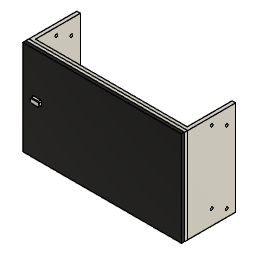
Radio Stack Avionics Template v10 (Autodesk Fusion 360 design; units mm, degrees)
Autodesk Fusion 360 part; units mm, degrees
sketch "Faceplate" plane through (0, 0, 0) normal (0, 1, 0) x (1, 0, 0) in component "Faceplate"
  line L0 (79.375, -47.3279) -> (-79.375, -47.3279)
  line L1 (-79.375, -47.3279) -> (-79.375, 47.3279)
  line L2 (-79.375, 47.3279) -> (79.375, 47.3279)
  line L3 (79.375, 47.3279) -> (79.375, -47.3279)
  line L4 (79.375, -47.3279) -> (-79.375, 47.3279) construction
  line L5 (-79.375, -47.3279) -> (79.375, 47.3279) construction
  line L6 (-65.5187, -6.373) -> (-65.5187, -0.373) construction
  arc A0 (-69.0187, -0.373) -> (-70.5187, -1.873) centre (-69.0187, -1.873) ccw
  line L7 (-62.0187, -0.373) -> (-69.0187, -0.373)
  line L8 (-70.5187, -1.873) -> (-70.5187, -4.873)
  line L9 (-60.5187, -4.873) -> (-60.5187, -1.873)
  arc A1 (-62.0187, -6.373) -> (-60.5187, -4.873) centre (-62.0187, -4.873) ccw
  line L10 (-69.0187, -6.373) -> (-62.0187, -6.373)
  arc A2 (-70.5187, -4.873) -> (-69.0187, -6.373) centre (-69.0187, -4.873) ccw
  arc A3 (-60.5187, -1.873) -> (-62.0187, -0.373) centre (-62.0187, -1.873) ccw
  line L11 (-77.2756, -49.1415) -> (67.16, -49.1415) construction
  line L12 (67.16, -49.1415) -> (67.16, -65.0937) construction
  line L13 (67.16, -65.0937) -> (-77.2756, -65.0937) construction
  line L14 (-77.2756, -65.0937) -> (-77.2756, -49.1415) construction
  point P0 (-65.5187, -3.373)
  dimension "d1" = 158.75
  dimension "d27" = 1.5
  dimension "d28" = 6
  dimension "d29" = 10
  dimension "d42" = 3
  constraint horizontal L0
  constraint perpendicular L0 L1
  constraint parallel L0 L2
  constraint parallel L1 L3
  constraint coincident L4 origin
  constraint coincident L5 origin
  constraint horizontal L10
  constraint vertical L9
  constraint horizontal L7
  constraint vertical L8
  constraint tangent A1 L10
  constraint tangent L9 A1
  constraint tangent L9 A3
  constraint tangent L7 A3
  constraint equal A1 A3
  constraint tangent A0 L7
  constraint tangent A0 L8
  constraint equal A0 A1
  constraint tangent L8 A2
  constraint tangent L10 A2
  constraint equal A1 A2
  constraint midpoint L6.start L10
  constraint midpoint L6.end L7
  constraint midpoint P0 L6
  measures "d1" distance of L1.end L2.end
  measures "d27" radius of A1
  measures "d28" distance of L7 L10
  measures "d29" distance of L8 L9
extrude "Extrude1" add sketch "Faceplate" against normal blind 3 makes body 1 in component "Faceplate"
ref_plane "WorkPlane1" through (0, 0, 0) normal (0, 1, 0) x (0, 0, 1) in component "Button Skirt Spacer"
sketch "Button Skirt (Gives buttons space behind faceplate)" plane through (0, 0, 0) normal (0, 1, 0) x (1, 0, 0) in component "Button Skirt Spacer"
  line L0 (-79.375, -47.3279) -> (-79.375, 47.3279)
  line L1 (79.375, -47.3279) -> (-79.375, -47.3279)
  line L2 (79.375, 47.3279) -> (79.375, -47.3279)
  line L3 (-79.375, 47.3279) -> (79.375, 47.3279)
  line L4 (-60.5187, -4.873) -> (-60.5187, -1.873)
  arc A0 (-62.0187, -6.373) -> (-60.5187, -4.873) centre (-62.0187, -4.873) ccw
  line L5 (-69.0187, -6.373) -> (-62.0187, -6.373)
  arc A1 (-70.5187, -4.873) -> (-69.0187, -6.373) centre (-69.0187, -4.873) ccw
  line L6 (-70.5187, -1.873) -> (-70.5187, -4.873)
  arc A2 (-69.0187, -0.373) -> (-70.5187, -1.873) centre (-69.0187, -1.873) ccw
  line L7 (-62.0187, -0.373) -> (-69.0187, -0.373)
  arc A3 (-60.5187, -1.873) -> (-62.0187, -0.373) centre (-62.0187, -1.873) ccw
  line L8 (-72.5187, -8.373) -> (-58.5187, -8.373)
  line L9 (-58.5187, -8.373) -> (-58.5187, 1.627)
  line L10 (-58.5187, 1.627) -> (-72.5187, 1.627)
  line L11 (-72.5187, 1.627) -> (-72.5187, -8.373)
  line L12 (-65.7771, -46.8251) -> (92.1912, -46.8251) construction
  line L13 (92.1912, -46.8251) -> (92.1912, -80.2756) construction
  line L14 (92.1912, -80.2756) -> (-65.7771, -80.2756) construction
  line L15 (-65.7771, -80.2756) -> (-65.7771, -46.8251) construction
  dimension "d37" = 2
  dimension "d38" = 2
  dimension "d39" = 2
  dimension "d40" = 2
  dimension "d41" = 3
  constraint horizontal L8
  constraint vertical L9
  constraint horizontal L10
  constraint vertical L11
  constraint horizontal L14
  measures "d37" distance of L4 L9
  measures "d38" distance of L5 L8
  measures "d39" distance of L6 L11
  measures "d40" distance of L7 L10
extrude "Extrude1'" add sketch "Button Skirt (Gives buttons space behind faceplate)" along normal blind 3 separate body contours L0 L1 L2 L3 | L4 A0 L5 A1 L6 A2 L7 A3 | L8 L9 L10 L11 makes body 2 in component "Button Skirt Spacer"
ref_plane "WorkPlane1" through (0, 3, 0) normal (0, 1, 0) x (0, 0, 1) in component "Non PCB Backing"
sketch "Sketch1" plane through (0, 3, 0) normal (0, 1, 0) x (1, 0, 0) in component "Non PCB Backing"
  line L0 (-79.375, -47.3279) -> (79.375, -47.3279)
  line L1 (-79.375, 47.3279) -> (-79.375, -47.3279)
  line L2 (79.375, 47.3279) -> (-79.375, 47.3279)
  line L3 (79.375, -47.3279) -> (79.375, 47.3279)
  arc A0 (-60.5187, -1.873) -> (-62.0187, -0.373) centre (-62.0187, -1.873) ccw construction
  line L4 (-62.0187, -0.373) -> (-69.0187, -0.373) construction
  arc A1 (-69.0187, -0.373) -> (-70.5187, -1.873) centre (-69.0187, -1.873) ccw construction
  line L5 (-70.5187, -1.873) -> (-70.5187, -4.873) construction
  arc A2 (-70.5187, -4.873) -> (-69.0187, -6.373) centre (-69.0187, -4.873) ccw construction
  line L6 (-69.0187, -6.373) -> (-62.0187, -6.373) construction
  arc A3 (-62.0187, -6.373) -> (-60.5187, -4.873) centre (-62.0187, -4.873) ccw construction
  line L7 (-60.5187, -4.873) -> (-60.5187, -1.873) construction
  line L8 (-79.375, 47.3279) -> (79.375, 47.3279)
  line L9 (79.375, 47.3279) -> (79.375, -47.3279)
  line L10 (79.375, -47.3279) -> (-79.375, -47.3279)
  line L11 (-79.375, -47.3279) -> (-79.375, 47.3279)
  line L12 (-69.0187, -4.873) -> (-62.0187, -1.873) construction
  line L13 (-62.4187, -0.123) -> (-68.6187, -0.123)
  line L14 (-68.6187, -0.123) -> (-68.6187, -6.623)
  line L15 (-68.6187, -6.623) -> (-62.4187, -6.623)
  line L16 (-62.4187, -6.623) -> (-62.4187, -0.123)
  line L17 (-62.4187, -0.123) -> (-68.6187, -6.623) construction
  line L18 (-68.6187, -0.123) -> (-62.4187, -6.623) construction
  line L19 (-152.6605, -47.3864) -> (11.8867, -47.2695) construction
  line L20 (11.8867, -47.2695) -> (11.9439, -127.8922) construction
  line L21 (11.9439, -127.8922) -> (-152.6032, -128.0091) construction
  line L22 (-152.6032, -128.0091) -> (-152.6605, -47.3864) construction
  line L23 (23.3274, -102.3824) -> (37.404, -102.3824)
  line L24 (37.404, -102.3824) -> (37.404, -92.7252)
  line L25 (37.404, -92.7252) -> (23.3274, -92.7252)
  line L26 (23.3274, -92.7252) -> (23.3274, -102.3824)
  line L27 (30.3657, -102.3824) -> (30.3657, -92.7252) construction
  line L28 (52.3764, -102.1676) -> (52.3764, -92.5104) construction
  line L29 (59.4147, -102.1676) -> (59.4147, -92.5104)
  line L30 (45.3381, -92.5104) -> (45.3381, -102.1676)
  line L31 (45.3381, -102.1676) -> (59.4147, -102.1676)
  line L32 (59.4147, -92.5104) -> (45.3381, -92.5104)
  line L33 (84.4147, -92.5104) -> (70.3381, -92.5104)
  line L34 (70.3381, -102.1676) -> (84.4147, -102.1676)
  line L35 (70.3381, -92.5104) -> (70.3381, -102.1676)
  line L36 (77.3764, -102.1676) -> (77.3764, -92.5104) construction
  line L37 (84.4147, -102.1676) -> (84.4147, -92.5104)
  line L38 (80.4764, -94.089) -> (74.2764, -94.089)
  line L39 (74.2764, -94.089) -> (74.2764, -100.589)
  line L40 (74.2764, -100.589) -> (80.4764, -100.589)
  line L41 (80.4764, -100.589) -> (80.4764, -94.089)
  line L42 (80.4764, -94.089) -> (74.2764, -100.589) construction
  line L43 (74.2764, -94.089) -> (80.4764, -100.589) construction
  line L44 (125.2683, -93.5274) -> (119.0683, -93.5274)
  line L45 (119.0683, -100.0274) -> (125.2683, -100.0274)
  line L46 (125.2683, -93.5274) -> (119.0683, -100.0274) construction
  line L47 (119.0683, -93.5274) -> (125.2683, -100.0274) construction
  line L48 (117.1683, -95.2774) -> (117.1683, -98.2774) construction
  arc A4 (118.6683, -93.7774) -> (117.1683, -95.2774) centre (118.6683, -95.2774) ccw construction
  line L49 (127.1683, -98.2774) -> (127.1683, -95.2774) construction
  line L50 (125.6683, -93.7774) -> (118.6683, -93.7774) construction
  arc A5 (127.1683, -95.2774) -> (125.6683, -93.7774) centre (125.6683, -95.2774) ccw construction
  arc A6 (125.6683, -99.7774) -> (127.1683, -98.2774) centre (125.6683, -98.2774) ccw construction
  arc A7 (117.1683, -98.2774) -> (118.6683, -99.7774) centre (118.6683, -98.2774) ccw construction
  line L51 (118.6683, -99.7774) -> (125.6683, -99.7774) construction
  line L52 (119.0683, -93.5274) -> (119.0683, -100.0274)
  line L53 (125.2683, -100.0274) -> (125.2683, -93.5274)
  line L54 (118.6683, -98.2774) -> (125.6683, -95.2774) construction
  line L55 (94.2764, -94.089) -> (94.2764, -100.589)
  line L56 (90.3381, -102.1676) -> (104.4147, -102.1676) construction
  line L57 (94.2764, -94.089) -> (100.4764, -100.589) construction
  line L58 (90.3381, -92.5104) -> (90.3381, -102.1676) construction
  line L59 (94.2764, -100.589) -> (100.4764, -100.589)
  line L60 (104.4147, -102.1676) -> (104.4147, -92.5104) construction
  line L61 (97.3764, -102.1676) -> (97.3764, -92.5104) construction
  line L62 (100.4764, -94.089) -> (94.2764, -94.089)
  line L63 (100.4764, -94.089) -> (94.2764, -100.589) construction
  line L64 (104.4147, -92.5104) -> (90.3381, -92.5104) construction
  line L65 (100.4764, -100.589) -> (100.4764, -94.089)
  point P0 (-65.5187, -3.373)
  point P1 (52.3764, -97.339)
  point P2 (77.3764, -97.339)
  point P3 (77.3764, -97.339)
  point P4 (122.1683, -96.7774)
  point P5 (97.3764, -97.339)
  point P6 (97.3764, -97.339)
  dimension "d45" = 6.2
  dimension "d46" = 6.5
  dimension "d47" = 3
  dimension "d48" = 6.2
  dimension "d49" = 6.5
  dimension "d50" = 6.2
  dimension "d51" = 6.5
  dimension "d52" = 6.2
  dimension "d53" = 6.5
  constraint coincident A2.centre L12.start
  constraint coincident A0.centre L12.end
  constraint horizontal L13
  constraint perpendicular L13 L14
  constraint parallel L13 L15
  constraint parallel L14 L16
  constraint coincident L17 P0
  constraint coincident L18 P0
  constraint midpoint L12 P0
  constraint horizontal L23
  constraint vertical L24
  constraint horizontal L25
  constraint vertical L26
  constraint midpoint L23 L27.start
  constraint midpoint L25 L27.end
  constraint horizontal L31
  constraint vertical L29
  constraint horizontal L32
  constraint vertical L30
  constraint midpoint L28.start L31
  constraint midpoint L28.end L32
  constraint midpoint L28 P1
  constraint horizontal L34
  constraint vertical L37
  constraint horizontal L33
  constraint vertical L35
  constraint midpoint L36.start L34
  constraint midpoint L36.end L33
  constraint midpoint P3 L36
  constraint horizontal L38
  constraint perpendicular L38 L39
  constraint parallel L38 L40
  constraint parallel L39 L41
  constraint coincident L42 P3
  constraint coincident L43 P3
  constraint coincident P3 P2
  constraint coincident A7.centre L54.start
  constraint coincident A5.centre L54.end
  constraint horizontal L44
  constraint perpendicular L44 L52
  constraint parallel L44 L45
  constraint parallel L52 L53
  constraint coincident P4 L46
  constraint coincident P4 L47
  constraint midpoint P4 L54
  constraint horizontal L56
  constraint vertical L60
  constraint horizontal L64
  constraint vertical L58
  constraint midpoint L61.start L56
  constraint midpoint L61.end L64
  constraint midpoint P6 L61
  constraint horizontal L62
  constraint perpendicular L55 L62
  constraint parallel L59 L62
  constraint parallel L55 L65
  constraint coincident P6 L63
  constraint coincident P6 L57
  constraint coincident P6 P5
  constraint coincident L10
  measures "d45" distance of L14.end L15.end
  measures "d46" distance of L13.end L14.end
  measures "d48" distance of L39.end L40.end
  measures "d49" distance of L38.end L39.end
  measures "d50" distance of L45.start L45.end
  measures "d51" distance of L45.start L44.end
  measures "d52" distance of L55.end L57.end
  measures "d53" distance of L55.end L55.start
extrude "Extrude1''" add sketch "Sketch1" along normal blind 3 separate body contours L0 L1 L2 L3 L8 L9 L10 L11 | L13 L14 L15 L16 makes body 3 in component "Non PCB Backing"
ref_plane "WorkPlane1" through (0, 3, 0) normal (0, 1, 0) x (0, 0, 1) in component "PCB Outline"
sketch "PCB Outline" plane through (0, 3, 0) normal (0, 1, 0) x (1, 0, 0) in component "PCB Outline"
  line L0 (-79.375, -47.3279) -> (79.375, -47.3279)
  line L1 (79.375, -47.3279) -> (79.375, 47.3279)
  line L2 (79.375, 47.3279) -> (-79.375, 47.3279)
  line L3 (-79.375, 47.3279) -> (-79.375, -47.3279)
extrude "Extrude1'''" add sketch "PCB Outline" along normal blind 1.5 separate body makes body 4 in component "PCB Outline"
ref_plane "WorkPlane1" through (0, 0, 0) normal (0, 1, 0) x (1, 0, 0) in component "Button Blank"
sketch "Top Profile" plane through (0, 0, 0) normal (0, 1, 0) x (1, 0, 0) in component "Button Blank"
  line L0 (-67.5508, -13.2161) -> (-67.5508, -10.2161) construction
  arc A0 (-66.0508, -8.7161) -> (-67.5508, -10.2161) centre (-66.0508, -10.2161) ccw construction
  line L1 (-66.0508, -8.7161) -> (-59.0508, -8.7161) construction
  arc A1 (-57.5508, -10.2161) -> (-59.0508, -8.7161) centre (-59.0508, -10.2161) ccw construction
  line L2 (-57.5508, -10.2161) -> (-57.5508, -13.2161) construction
  arc A2 (-59.0508, -14.7161) -> (-57.5508, -13.2161) centre (-59.0508, -13.2161) ccw construction
  line L3 (-59.0508, -14.7161) -> (-66.0508, -14.7161) construction
  arc A3 (-67.5508, -13.2161) -> (-66.0508, -14.7161) centre (-66.0508, -13.2161) ccw construction
  arc A4 (-68.8008, -13.2161) -> (-66.0508, -15.9661) centre (-66.0508, -13.2161) ccw
  line L4 (-59.0508, -15.9661) -> (-66.0508, -15.9661)
  arc A5 (-59.0508, -15.9661) -> (-56.3008, -13.2161) centre (-59.0508, -13.2161) ccw
  line L5 (-56.3008, -10.2161) -> (-56.3008, -13.2161)
  arc A6 (-56.3008, -10.2161) -> (-59.0508, -7.4661) centre (-59.0508, -10.2161) ccw
  line L6 (-66.0508, -7.4661) -> (-59.0508, -7.4661)
  arc A7 (-66.0508, -7.4661) -> (-68.8008, -10.2161) centre (-66.0508, -10.2161) ccw
  line L7 (-68.8008, -13.2161) -> (-68.8008, -10.2161)
  line L8 (-59.0508, -14.2161) -> (-66.0508, -14.2161)
  arc A8 (-67.0508, -13.2161) -> (-66.0508, -14.2161) centre (-66.0508, -13.2161) ccw
  line L9 (-67.0508, -13.2161) -> (-67.0508, -10.2161)
  arc A9 (-66.0508, -9.2161) -> (-67.0508, -10.2161) centre (-66.0508, -10.2161) ccw
  line L10 (-66.0508, -9.2161) -> (-59.0508, -9.2161)
  arc A10 (-58.0508, -10.2161) -> (-59.0508, -9.2161) centre (-59.0508, -10.2161) ccw
  line L11 (-58.0508, -10.2161) -> (-58.0508, -13.2161)
  arc A11 (-59.0508, -14.2161) -> (-58.0508, -13.2161) centre (-59.0508, -13.2161) ccw
  line L12 (-66.0508, -13.2161) -> (-59.0508, -10.2161) construction
  line L13 (-79.375, -47.3279) -> (-79.375, 47.3279)
  line L14 (-79.375, 47.3279) -> (79.375, 47.3279)
  line L15 (79.375, 47.3279) -> (79.375, -47.3279)
  line L16 (79.375, -47.3279) -> (-79.375, -47.3279)
  line L17 (-69.0187, -6.373) -> (-62.0187, -6.373) construction
  arc A12 (-62.0187, -6.373) -> (-60.5187, -4.873) centre (-62.0187, -4.873) ccw construction
  line L18 (-60.5187, -4.873) -> (-60.5187, -1.873) construction
  arc A13 (-60.5187, -1.873) -> (-62.0187, -0.373) centre (-62.0187, -1.873) ccw construction
  line L19 (-62.0187, -0.373) -> (-69.0187, -0.373) construction
  arc A14 (-69.0187, -0.373) -> (-70.5187, -1.873) centre (-69.0187, -1.873) ccw construction
  line L20 (-70.5187, -1.873) -> (-70.5187, -4.873) construction
  arc A15 (-70.5187, -4.873) -> (-69.0187, -6.373) centre (-69.0187, -4.873) ccw construction
  line L21 (-62.0187, -0.873) -> (-69.0187, -0.873)
  arc A16 (-69.0187, -0.873) -> (-70.0187, -1.873) centre (-69.0187, -1.873) ccw
  line L22 (-70.0187, -1.873) -> (-70.0187, -4.873)
  arc A17 (-70.0187, -4.873) -> (-69.0187, -5.873) centre (-69.0187, -4.873) ccw
  line L23 (-69.0187, -5.873) -> (-62.0187, -5.873)
  arc A18 (-62.0187, -5.873) -> (-61.0187, -4.873) centre (-62.0187, -4.873) ccw
  line L24 (-61.0187, -4.873) -> (-61.0187, -1.873)
  arc A19 (-61.0187, -1.873) -> (-62.0187, -0.873) centre (-62.0187, -1.873) ccw
  line L25 (-59.2687, -4.873) -> (-59.2687, -1.873)
  arc A20 (-59.2687, -1.873) -> (-62.0187, 0.877) centre (-62.0187, -1.873) ccw
  line L26 (-62.0187, 0.877) -> (-69.0187, 0.877)
  arc A21 (-69.0187, 0.877) -> (-71.7687, -1.873) centre (-69.0187, -1.873) ccw
  line L27 (-71.7687, -1.873) -> (-71.7687, -4.873)
  arc A22 (-71.7687, -4.873) -> (-69.0187, -7.623) centre (-69.0187, -4.873) ccw
  line L28 (-69.0187, -7.623) -> (-62.0187, -7.623)
  arc A23 (-62.0187, -7.623) -> (-59.2687, -4.873) centre (-62.0187, -4.873) ccw
  point P0 (-62.5508, -11.7161)
  dimension "d95_2_1" = 1.25
  dimension "d96_2_1" = 0.5
  dimension "d16_1" = -0.5
  dimension "d17_1" = 1.25
  constraint coincident A3.centre A4.centre
  constraint coincident A1.centre A6.centre
  constraint midpoint L12 P0
extrude "Extrude1''''" add sketch "Top Profile" along normal blind 1 separate body contours L6 A7 L25 A20 L26 A21 L27 A22 L28 A23 | L6 A7 L28 A23 | L21 A16 L22 A17 L23 A18 L24 A19 makes body 5 in component "Button Blank"
extrude "Extrude2" add sketch "Top Profile" against normal up to surface (5.5 mm away) contours L21 A16 L22 A17 L23 A18 L24 A19 bodies 5 in component "Button Blank"
fillet "Fillet1" radius 0.5 8 edges at (-70.0187, -5.5, 3.373) (-69.7258, -5.5, 5.5801) (-65.5187, -5.5, 5.873) (-61.3116, -5.5, 5.5801) (-61.0187, -5.5, 3.373) (-61.3116, -5.5, 1.1659) (-65.5187, -5.5, 0.873) (-69.7258, -5.5, 1.1659) on bodies 5 in component "Button Blank"
sketch "Sketch2" plane through (0, 6, 0) normal (0, 1, 0) x (-1, 0, 0) in component "Non PCB Backing"
  line L0 (-79.375, 47.3279) -> (-79.375, -47.3279)
  line L1 (-79.375, -47.3279) -> (79.375, -47.3279)
  line L2 (79.375, -47.3279) -> (79.375, 47.3279)
  line L3 (79.375, 47.3279) -> (-79.375, 47.3279)
  line L4 (-75.875, 47.3279) -> (-75.875, -47.3279)
  line L5 (75.875, 47.3279) -> (75.875, -47.3279)
  dimension "d20" = 3.5
  dimension "d21" = 3.5
  constraint perpendicular L3 L4
  constraint coincident L1 L5.end
  constraint perpendicular L1 L5
  constraint coincident L3 L5.start
  constraint coincident L3 L4.start
  constraint coincident L1 L4.end
  measures "d20" distance of L0 L4
  measures "d21" distance of L2 L5
extrude "Extrude2'" add sketch "Sketch2" along normal blind 45 contours L0 L1 L3 L4 | L1 L2 L3 L5 bodies 3 in component "Non PCB Backing"
sketch "Sketch3" plane through (-79.375, 0, 0) normal (-1, 0, 0) x (0, -1, 0) in component "Non PCB Backing"
  line L0 (-3, -47.3279) -> (-3, 47.3279)
  line L1 (-3, 47.3279) -> (-51, 47.3279)
  line L2 (-51, 47.3279) -> (-51, -47.3279)
  line L3 (-51, -47.3279) -> (-3, -47.3279)
  circle A0 centre (-27, 39.8279) radius 1.4
  circle A1 centre (-27, -32.3279) radius 1.4
  circle A2 centre (-42, 32.3279) radius 1.4
  circle A3 centre (-42, -39.8279) radius 1.4
  line L4 (3, 47.3279) -> (3, -47.3279)
  dimension "d24" = 2.8
  dimension "d25" = 72.1559
  dimension "d26" = 94.6559
  dimension "d30" = 72.1559
  dimension "d31" = 15
  dimension "d32" = 30
  dimension "d33" = 15
  dimension "d34" = 7.5
  constraint equal A1 A3
  constraint equal A2 A3
  constraint equal A0 A2
  constraint vertical A0.centre A1.centre
  constraint vertical A2.centre A3.centre
  measures "d24" diameter of A0
  measures "d25" distance of A0.centre A1.centre
  measures "d26" distance of L1.end L2.end
  measures "d30" distance of A2.centre A3.centre
  measures "d31" distance of L1 A2.centre
  measures "d32" distance of A0.centre L4
  measures "d33" horizontal distance of A0.centre A2.centre
  measures "d34" distance of L1 A0.centre
ref_plane "WorkPlane1" through (0, 0, 0) normal (0, 1, 0) x (1, 0, 0) in component "Blank Button"
sketch "Top Profile (2)" plane through (0, 0, 0) normal (0, 1, 0) x (1, 0, 0) in component "Blank Button"
  line L0 (-67.5508, -13.2161) -> (-67.5508, -10.2161) construction
  arc A0 (-66.0508, -8.7161) -> (-67.5508, -10.2161) centre (-66.0508, -10.2161) ccw construction
  line L1 (-66.0508, -8.7161) -> (-59.0508, -8.7161) construction
  arc A1 (-57.5508, -10.2161) -> (-59.0508, -8.7161) centre (-59.0508, -10.2161) ccw construction
  line L2 (-57.5508, -10.2161) -> (-57.5508, -13.2161) construction
  arc A2 (-59.0508, -14.7161) -> (-57.5508, -13.2161) centre (-59.0508, -13.2161) ccw construction
  line L3 (-59.0508, -14.7161) -> (-66.0508, -14.7161) construction
  arc A3 (-67.5508, -13.2161) -> (-66.0508, -14.7161) centre (-66.0508, -13.2161) ccw construction
  arc A4 (-68.8008, -13.2161) -> (-66.0508, -15.9661) centre (-66.0508, -13.2161) ccw
  line L4 (-59.0508, -15.9661) -> (-66.0508, -15.9661)
  arc A5 (-59.0508, -15.9661) -> (-56.3008, -13.2161) centre (-59.0508, -13.2161) ccw
  line L5 (-56.3008, -10.2161) -> (-56.3008, -13.2161)
  arc A6 (-56.3008, -10.2161) -> (-59.0508, -7.4661) centre (-59.0508, -10.2161) ccw
  line L6 (-66.0508, -7.4661) -> (-59.0508, -7.4661)
  arc A7 (-66.0508, -7.4661) -> (-68.8008, -10.2161) centre (-66.0508, -10.2161) ccw
  line L7 (-68.8008, -13.2161) -> (-68.8008, -10.2161)
  line L8 (-59.0508, -14.2161) -> (-66.0508, -14.2161)
  arc A8 (-67.0508, -13.2161) -> (-66.0508, -14.2161) centre (-66.0508, -13.2161) ccw
  line L9 (-67.0508, -13.2161) -> (-67.0508, -10.2161)
  arc A9 (-66.0508, -9.2161) -> (-67.0508, -10.2161) centre (-66.0508, -10.2161) ccw
  line L10 (-66.0508, -9.2161) -> (-59.0508, -9.2161)
  arc A10 (-58.0508, -10.2161) -> (-59.0508, -9.2161) centre (-59.0508, -10.2161) ccw
  line L11 (-58.0508, -10.2161) -> (-58.0508, -13.2161)
  arc A11 (-59.0508, -14.2161) -> (-58.0508, -13.2161) centre (-59.0508, -13.2161) ccw
  line L12 (-66.0508, -13.2161) -> (-59.0508, -10.2161) construction
  line L13 (-79.375, -47.3279) -> (-79.375, 47.3279)
  line L14 (-79.375, 47.3279) -> (79.375, 47.3279)
  line L15 (79.375, 47.3279) -> (79.375, -47.3279)
  line L16 (79.375, -47.3279) -> (-79.375, -47.3279)
  line L17 (-69.0187, -6.373) -> (-62.0187, -6.373) construction
  arc A12 (-62.0187, -6.373) -> (-60.5187, -4.873) centre (-62.0187, -4.873) ccw construction
  line L18 (-60.5187, -4.873) -> (-60.5187, -1.873) construction
  arc A13 (-60.5187, -1.873) -> (-62.0187, -0.373) centre (-62.0187, -1.873) ccw construction
  line L19 (-62.0187, -0.373) -> (-69.0187, -0.373) construction
  arc A14 (-69.0187, -0.373) -> (-70.5187, -1.873) centre (-69.0187, -1.873) ccw construction
  line L20 (-70.5187, -1.873) -> (-70.5187, -4.873) construction
  arc A15 (-70.5187, -4.873) -> (-69.0187, -6.373) centre (-69.0187, -4.873) ccw construction
  line L21 (-62.0187, -0.873) -> (-69.0187, -0.873)
  arc A16 (-69.0187, -0.873) -> (-70.0187, -1.873) centre (-69.0187, -1.873) ccw
  line L22 (-70.0187, -1.873) -> (-70.0187, -4.873)
  arc A17 (-70.0187, -4.873) -> (-69.0187, -5.873) centre (-69.0187, -4.873) ccw
  line L23 (-69.0187, -5.873) -> (-62.0187, -5.873)
  arc A18 (-62.0187, -5.873) -> (-61.0187, -4.873) centre (-62.0187, -4.873) ccw
  line L24 (-61.0187, -4.873) -> (-61.0187, -1.873)
  arc A19 (-61.0187, -1.873) -> (-62.0187, -0.873) centre (-62.0187, -1.873) ccw
  line L25 (-59.2687, -4.873) -> (-59.2687, -1.873)
  arc A20 (-59.2687, -1.873) -> (-62.0187, 0.877) centre (-62.0187, -1.873) ccw
  line L26 (-62.0187, 0.877) -> (-69.0187, 0.877)
  arc A21 (-69.0187, 0.877) -> (-71.7687, -1.873) centre (-69.0187, -1.873) ccw
  line L27 (-71.7687, -1.873) -> (-71.7687, -4.873)
  arc A22 (-71.7687, -4.873) -> (-69.0187, -7.623) centre (-69.0187, -4.873) ccw
  line L28 (-69.0187, -7.623) -> (-62.0187, -7.623)
  arc A23 (-62.0187, -7.623) -> (-59.2687, -4.873) centre (-62.0187, -4.873) ccw
  point P0 (-62.5508, -11.7161)
  dimension "d95_2_1_1" = 1.25
  dimension "d96_2_1_1" = 0.5
  dimension "d16_1_1" = -0.5
  dimension "d17_1_1" = 1.25
  constraint coincident A3.centre A4.centre
  constraint coincident A1.centre A6.centre
  constraint midpoint L12 P0
extrude "Extrude1'''''" add sketch "Top Profile (2)" along normal blind 1 separate body contours L6 A7 L25 A20 L26 A21 L27 A22 L28 A23 | L6 A7 L28 A23 | L21 A16 L22 A17 L23 A18 L24 A19 makes body 6 in component "Blank Button"
extrude "Extrude2''" add sketch "Top Profile (2)" against normal up to surface (5.5 mm away) contours L21 A16 L22 A17 L23 A18 L24 A19 bodies 6 in component "Blank Button"
fillet "Fillet1'" radius 0.5 8 edges at (-70.0187, -5.5, 3.373) (-69.7258, -5.5, 5.5801) (-65.5187, -5.5, 5.873) (-61.3116, -5.5, 5.5801) (-61.0187, -5.5, 3.373) (-61.3116, -5.5, 1.1659) (-65.5187, -5.5, 0.873) (-69.7258, -5.5, 1.1659) on bodies 6 in component "Blank Button"
sketch "Text" plane through (0, -5.5, 0) normal (0, -1, 0) x (1, 0, 0) in component "Blank Button"
  line L0 (-69.5187, 2.3109) -> (-61.5187, 2.3109) construction
  line L1 (-61.5187, 2.3109) -> (-61.5187, 4.4352) construction
  line L2 (-61.5187, 4.4352) -> (-69.5187, 4.4352) construction
  line L3 (-69.5187, 4.4352) -> (-69.5187, 2.3109) construction
  line L4 (-69.5187, 4.873) -> (-69.5187, 1.873)
  arc A0 (-69.5187, 1.873) -> (-69.0187, 1.373) centre (-69.0187, 1.873) ccw
  line L5 (-69.0187, 1.373) -> (-62.0187, 1.373)
  arc A1 (-62.0187, 1.373) -> (-61.5187, 1.873) centre (-62.0187, 1.873) ccw
  line L6 (-61.5187, 1.873) -> (-61.5187, 4.873)
  arc A2 (-61.5187, 4.873) -> (-62.0187, 5.373) centre (-62.0187, 4.873) ccw
  line L7 (-62.0187, 5.373) -> (-69.0187, 5.373)
  arc A3 (-69.0187, 5.373) -> (-69.5187, 4.873) centre (-69.0187, 4.873) ccw
  dimension "d134_1_1_1" = 3.5
  constraint midpoint L6
  constraint midpoint L4
extrude "Extrude3" [suppressed] in component "Blank Button"
sketch "Front" plane through (0, 4.5, 0) normal (0, 1, 0) x (-1, 0, 0) in component "PCB Radio Stack Mount"
  line L0 (79.375, -47.3279) -> (79.375, 47.3279)
  line L1 (79.375, 47.3279) -> (-79.375, 47.3279)
  line L2 (-79.375, 47.3279) -> (-79.375, -47.3279)
  line L3 (-79.375, -47.3279) -> (79.375, -47.3279)
  line L4 (-66.875, 47.3279) -> (-66.875, -47.3279)
  line L5 (66.875, 47.3279) -> (66.875, -47.3279)
  line L6 (-75.875, 47.3279) -> (-75.875, -47.3279)
  line L7 (75.875, 47.3279) -> (75.875, 43.9611)
  line L8 (75.875, 43.9611) -> (75.875, -47.3279)
  dimension "d54" = 12.5
  dimension "d55" = 12.5
  dimension "d56" = 3.5
  dimension "d57" = 3.5
  constraint coincident L1 L4.start
  constraint coincident L3 L4.end
  constraint perpendicular L3 L4
  constraint perpendicular L3 L5
  constraint coincident L3 L5.end
  constraint coincident L1 L5.start
  constraint coincident L1 L6.start
  constraint coincident L3 L6.end
  constraint perpendicular L3 L6
  constraint coincident L1 L7.start
  constraint perpendicular L1 L7
  constraint coincident L3 L8.end
  constraint perpendicular L3 L8
  measures "d54" distance of L2 L4
  measures "d55" distance of L0 L5
  measures "d56" distance of L0 L8
  measures "d57" distance of L2 L6
extrude "Extrude1''''''" add sketch "Front" along normal blind 45 separate body contours L0 L1 L3 L7 L8 | L1 L2 L3 L6 makes body 7 at (79.375, 19.5, 15.776) makes body 8 at (-75.875, 19.5, 15.776) in component "PCB Radio Stack Mount"
extrude "Extrude2'''" add sketch "Front" along normal blind 3 contours L1 L3 L5 L7 L8 | L1 L3 L4 L6 bodies 7 8 in component "PCB Radio Stack Mount"
extrude "Extrude3'" cut sketch "Sketch3" against normal through all contours A0 | A1 | A2 | A3 bodies 3 in component "Non PCB Backing"
extrude "Extrude3''" cut sketch "Sketch3" against normal through all contours A0 | A1 | A2 | A3 bodies 7 8 in component "PCB Radio Stack Mount"
copy_body "CutPasteBodies1" bodies 5 removing the originals makes body 9 in component "Buttons"
sketch "Instructions" plane through (0, -5.5, 0) normal (0, -1, 0) x (1, 0, 0) in component "Buttons"
  line L0 (-69.5187, 4.873) -> (-69.5187, 1.873)
  arc A0 (-69.5187, 1.873) -> (-69.0187, 1.373) centre (-69.0187, 1.873) ccw
  line L1 (-69.0187, 1.373) -> (-62.0187, 1.373)
  arc A1 (-62.0187, 1.373) -> (-61.5187, 1.873) centre (-62.0187, 1.873) ccw
  line L2 (-61.5187, 1.873) -> (-61.5187, 4.873)
  arc A2 (-61.5187, 4.873) -> (-62.0187, 5.373) centre (-62.0187, 4.873) ccw
  line L3 (-62.0187, 5.373) -> (-69.0187, 5.373)
  arc A3 (-69.0187, 5.373) -> (-69.5187, 4.873) centre (-69.0187, 4.873) ccw
  line L4 (-125.6395, -34.5454) -> (-63.7106, -34.5454) construction
  line L5 (-63.7106, -34.5454) -> (-63.7106, 32.2808) construction
  line L6 (-63.7106, 32.2808) -> (-125.6395, 32.2808) construction
  line L7 (-125.6395, 32.2808) -> (-125.6395, -34.5454) construction
  dimension "d64" = 3
component "Faceplate" placed x (1, 0, 0) y (0, 1, 0) z (0, 0, 1) at (0, 0, 0)
component "Button Skirt Spacer" placed x (1, 0, 0) y (0, 1, 0) z (0, 0, 1) at (0, 0, 0)
component "Non PCB Backing" placed x (1, 0, 0) y (0, 1, 0) z (0, 0, 1) at (0, 0, 0)
component "PCB Outline" placed x (1, 0, 0) y (0, 1, 0) z (0, 0, 1) at (0, 0, 0)
component "PCB Radio Stack Mount" placed x (1, 0, 0) y (0, 1, 0) z (0, 0, 1) at (0, 0, 0)
component "Electronics" placed x (1, 0, 0) y (0, 1, 0) z (0, 0, 1) at (0, 0, 0)
component "Buttons" placed x (1, 0, 0) y (0, 1, 0) z (0, 0, 1) at (0, 0, 0)
component "Blank Button" placed x (1, 0, 0) y (0, 1, 0) z (0, 0, 1) at (0, 0, 0) in component "Buttons"
equation "d1 = 6.25 \""
equation "TextExtrudeDist = 1 mm"
equation "d21 = d20"
equation "d25 = d26 - 22.5 mm"
equation "d30 = d26 - 22.5 mm"
equation "d135_1_1_1 = TextExtrudeDist"
equation "d37 = d38"
equation "d39 = d38"
equation "d40 = d38"
equation "ButtonX = 6.2 mm"
equation "ButtonY = 6.5 mm"
equation "d45 = ButtonX"
equation "d46 = ButtonY"
equation "d48 = ButtonX"
equation "d49 = ButtonY"
equation "d50 = ButtonX"
equation "d51 = ButtonY"
equation "d52 = ButtonX"
equation "d53 = ButtonY"
equation "d55 = d54"
equation "d56 = d57"
named bodies: "No PCB Backing", "Button to Rectangle Pattern"
